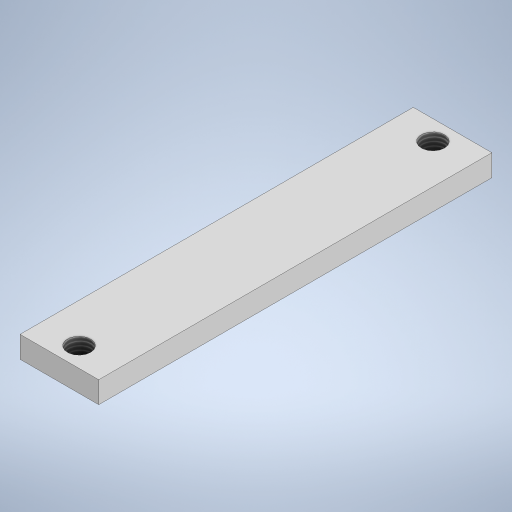
# Autodesk Inventor part: CB
Saved by Autodesk Inventor 2023 (Build 270158000, 158)
## iProperties
Created: 2022-10-24
Part Number: CB
Material: Generic
Document SubType Name: Modeling
Designer: User
Density: 1 g/cm^3
Appearance: Default
Author: User
Autodesk Inventor part; units mm, degrees
ref_plane "YZ Plane" through (0, 0, 0) normal (1, 0, 0) x (0, 1, 0)
ref_plane "XZ Plane" through (0, 0, 0) normal (0, 1, 0) x (-1, 0, 0)
ref_plane "XY Plane" through (0, 0, 0) normal (0, 0, 1) x (1, 0, 0)
sketch "Sketch1" plane through (0, 0, 0) normal (0, 1, 0) x (-1, 0, 0)
  line L0 (0, 0) -> (0, -100)
  line L1 (0, -100) -> (20, -100)
  line L2 (20, -100) -> (20, 0)
  line L3 (20, 0) -> (0, 0)
  point P0 (10, -5)
  point P1 (10, -95)
  dimension "d0" = 100
  dimension "d1" = 20
  dimension "d2" = 90
  dimension "d3" = 5
  constraints: 8 end point, 2 vertical, 1 horizontal, 1 perpendicular
  measures "d0" distance of L0.start L0.end
  measures "d1" distance of L0.end L1.end
  measures "d2" distance of point (10, -95) point (10, -5)
  measures "d3" distance from line of L3 point (10, -5)
extrude "Extrusion1" add sketch "Sketch1" along normal blind 5.5
hole "Hole1" at (-10, 0, -5) at (-10, 0, -95) direction (0, 1, 0) diameter 5.9175 depth 19.1 tip angle 118 thread size "M7x1" class "6H" standard "ANSI Metric M Profile"
body "Solid1"
